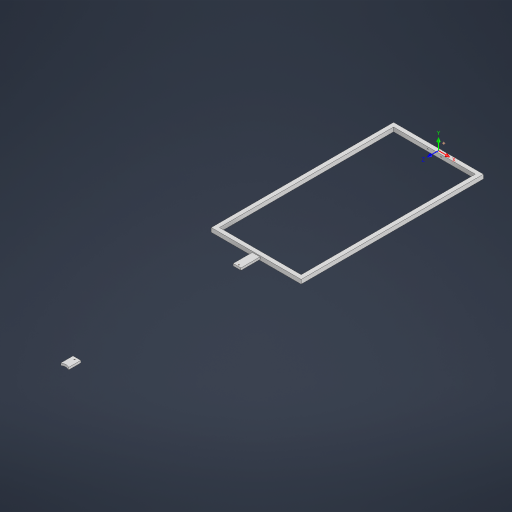
# Autodesk Inventor part: Marco
Saved by Autodesk Inventor 2024 (Build 280153000, 153)
## iProperties
Created: 2023-05-13
Part Number: Marco
Material: Genérico
Document SubType Name: Modeling
Designer: javie
Density: 1 g/cm^3
Appearance: Valor por defecto
Author: javie
Autodesk Inventor part; units mm, degrees
ref_plane "YZ Plane" through (0, 0, 0) normal (1, 0, 0) x (0, 1, 0)
ref_plane "XZ Plane" through (0, 0, 0) normal (0, 1, 0) x (-1, 0, 0)
sketch "Boceto2" plane through (0, 0, 0) normal (0, 1, 0) x (-1, 0, 0)
  line L0 (350, 0) -> (-350, 0)
  line L1 (-350, 0) -> (-350, 1000)
  line L2 (-120, 1500) -> (80, 1500)
  line L3 (350, 1000) -> (350, 0)
  line L4 (80, 1000) -> (80, 1500)
  line L5 (-120, 1000) -> (-120, 1500)
  line L6 (350, 1000) -> (80, 1000)
  line L7 (-120, 1000) -> (-350, 1000)
  arc A0 (-28.4, 1398.4243) -> (0, 1398.4243) centre (-14.2, 1419) ccw
  line L8 (-28.4, 1398.4243) -> (-28.4, 698.4243)
  line L9 (-28.4, 698.4243) -> (0, 698.4243)
  line L10 (0, 698.4243) -> (0, 1398.4243)
  line L11 (150, 698.4243) -> (-178.4, 698.4243)
  line L12 (-178.4, 698.4243) -> (-178.4, 32.4243)
  line L13 (-178.4, 32.4243) -> (150, 32.4243)
  line L14 (150, 32.4243) -> (150, 698.4243)
  point P0 (-14.2, 698.4243)
  dimension "d16" = 105.8
  dimension "d17" = 81
  dimension "d18" = 700
  dimension "d19" = 28.4
  dimension "d21" = 666
  dimension "d22" = 150
  dimension "d23" = 150
  dimension "d24" = 0
  constraints: 30 end point, 6 parallel, 5 perpendicular, 2 horizontal, 2 point on circle, 1 centre point, 1 midpoint
  measures "d16" distance from line of L5 A0.centre
  measures "d17" distance from line of L2 A0.centre
  measures "d18" distance of L8.start L8.end
  measures "d19" distance between parallel lines of L8 L10
  measures "d21" distance of L12.end L11.end
  measures "d22" distance between parallel lines of L10 L14
  measures "d23" distance between parallel lines of L12 L8
  measures "d24" distance from line of point (-14.2, 698.424) L11
extrude "Extrusión1" add sketch "Boceto2" along normal mid plane 15 contours L9 L11 L14 L13 L12
extrude "Extrusión2" add sketch "Boceto2" along normal mid plane 8 contours A0 L10 L9 L8
sketch "Boceto3" plane through (0, -7.5, 0) normal (0, -1, 0) x (1, 0, 0)
  line L0 (-150, 698.4243) -> (178.4, 698.4243) projected
  line L1 (178.4, 698.4243) -> (178.4, 32.4243) projected
  line L2 (-150, 698.4243) -> (178.4, 698.4243)
  line L3 (178.4, 698.4243) -> (178.4, 32.4243)
  line L4 (178.4, 32.4243) -> (-150, 32.4243)
  line L5 (-150, 32.4243) -> (-150, 698.4243)
  line L6 (-135, 683.4243) -> (163.4, 683.4243)
  line L7 (163.4, 683.4243) -> (163.4, 47.4243)
  line L8 (163.4, 47.4243) -> (-135, 47.4243)
  line L9 (-135, 47.4243) -> (-135, 683.4243)
  point P0 (0, 0)
  dimension "d29" = 15
  dimension "d30" = 15
  dimension "d31" = 15
  dimension "d32" = 15
  dimension "d49" = 666
  constraints: 16 end point, 4 parallel, 2 horizontal, 2 perpendicular
  measures "d29" distance between parallel lines of L5 L9
  measures "d30" distance between parallel lines of L1 L7
  measures "d31" distance between parallel lines of L4 L8
  measures "d32" distance between parallel lines of L0 L6
  measures "d49" distance of L0.end L1.end
extrude "Extrusión3" cut sketch "Boceto3" against normal blind 15 contours L6 L7 L8 L9
sketch "Boceto4" plane through (0, -4, 0) normal (0, -1, 0) x (1, 0, 0)
  line L0 (0, 698.4243) -> (0, 1398.4243) projected
  line L1 (28.4, 1398.4243) -> (28.4, 698.4243) projected
  line L2 (0, 768.4243) -> (28.4, 768.4243)
  line L3 (28.4, 768.4243) -> (28.4, 1353.4243)
  line L4 (28.4, 1353.4243) -> (0, 1353.4243)
  line L5 (0, 1353.4243) -> (0, 768.4243)
  line L6 (178.4, 698.4243) -> (-150, 698.4243) projected
  circle A0 centre (14.2, 1362.1792) radius 2
  circle A1 centre (14.2, 761.8658) radius 2
  point P0 (0, 0)
  point P1 (14.2, 698.4243)
  point P2 (14.2, 1353.4243)
  point P3 (0, 1353.4243)
  dimension "d35" = 70
  dimension "d36" = 45
  dimension "d37" = 4
  dimension "d38" = 4
  constraints: 8 end point, 2 centre point, 2 midpoint, 2 parallel, 2 point on line, 1 horizontal, 1 perpendicular
  measures "d35" distance from line of point (14.2, 698.424) L2
  measures "d36" vertical distance of point (14.2, 1353.424) L1.start
  measures "d37" diameter of A0
  measures "d38" diameter of A1
extrude "Extrusión4" cut sketch "Boceto4" against normal blind 15 contours L0 L4 L1 L2 | A0 | A1
ref_plane "Plano de trabajo1" through (0, 0, 0) normal (0, -1, 0) x (1, 0, 0)
sketch "Boceto5" plane through (0, 0, 0) normal (0, -1, 0) x (1, 0, 0)
  circle A0 centre (14.2, 1362.1792) radius 2
  point P0 (0, 0)
  point P1 (14.2, 761.8658)
  point P2 (14.2, 759.8658)
  point P3 (14.2, 763.8658)
  point P4 (14.2, 1364.1792)
  point P5 (14.2, 1360.1792)
  constraints: 2 point on circle, 1 centre point, 1 coincident
sketch "Boceto6" plane through (178.4, 7.5, 32.4243) normal (0, 0, -1) x (-1, 0, 0)
  line L0 (0, -15) -> (0, 0) projected
  line L1 (0, 0) -> (328.4, 0) projected
  point P0 (178.4, -7.5)
  point P1 (164.2, -7.5)
  point P2 (0, -7.5)
  dimension "d41" = 164.2
  dimension "d42" = 7.5
  constraints: 1 midpoint
  measures "d41" distance of point (0, -7.5) point (164.2, -7.5)
  measures "d42" distance from line of L1 point (164.2, -7.5)
sketch "Boceto7" plane through (-135, -7.5, 47.4243) normal (0, 0, 1) x (1, 0, 0)
  circle A0 centre (124.2, 7.5) radius 2
  circle A1 centre (174.2, 7.5) radius 2
  line L0 (0, 0) -> (0, 15) projected
  line L1 (0, 15) -> (298.4, 15) projected
  point P0 (135, 7.5)
  point P1 (0, 7.5)
  dimension "d50" = 4
  dimension "d51" = 4
  dimension "d52" = 124.2
  dimension "d53" = 174.2
  dimension "d54" = 50
  dimension "d55" = 7.5
  constraints: 2 centre point, 1 midpoint
  measures "d50" diameter of A0
  measures "d51" diameter of A1
  measures "d52" distance from line of A0.centre L0
  measures "d53" distance of point (0, 7.5) A1.centre
  measures "d54" distance of A1.centre A0.centre
  measures "d55" distance from line of L1 A0.centre
extrude "Extrusión5" cut sketch "Boceto7" against normal blind 10
